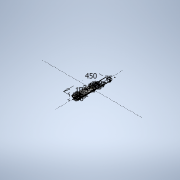
# Autodesk Inventor part: MoreFunComing-EnlosureEquipmentPanel
Saved by Autodesk Inventor 2021 (Build 250183000, 183)
## iProperties
Created: 2021-01-09
Part Number: MoreFunComing-EnlosureEquipmentPanel
Material: Generic
Document SubType Name: Modeling
Designer: incep
Density: 1 g/cm^3
Appearance: Default
Author: incep
Autodesk Inventor part; units mm, degrees
ref_plane "YZ Plane" through (0, 0, 0) normal (1, 0, 0) x (0, 1, 0)
ref_plane "XZ Plane" through (0, 0, 0) normal (0, 1, 0) x (-1, 0, 0)
ref_plane "XY Plane" through (0, 0, 0) normal (0, 0, 1) x (1, 0, 0)
sketch "Sketch1" plane through (0, 0, 0) normal (0, 1, 0) x (-1, 0, 0)
  line L0 (37.5, -225) -> (-37.5, -225)
  line L1 (-37.5, -225) -> (-37.5, 225)
  line L2 (-37.5, 225) -> (37.5, 225)
  line L3 (37.5, 225) -> (37.5, -225)
  line L4 (673.3706, 0) -> (-691.4675, 0) construction
  line L5 (0, 481.6336) -> (0, -423.6346) construction
  line L6 (31.5, -219) -> (-31.5, -219) construction
  line L7 (-31.5, -219) -> (-31.5, 219) construction
  line L8 (-31.5, 219) -> (31.5, 219) construction
  line L9 (31.5, 219) -> (31.5, -219) construction
  line L10 (34.5, -222) -> (-34.5, -222) construction
  line L11 (-34.5, -222) -> (-34.5, 222) construction
  line L12 (-34.5, 222) -> (34.5, 222) construction
  line L13 (34.5, 222) -> (34.5, -222) construction
  line L14 (14.5, 154.5) -> (-14.5, 154.5)
  line L15 (-14.5, 154.5) -> (-14.5, 211.5)
  line L16 (-14.5, 211.5) -> (14.5, 211.5)
  line L17 (14.5, 211.5) -> (14.5, 154.5)
  line L18 (50.1754, 183) -> (-68.7918, 183) construction
  circle A0 centre (20, 183) radius 1.5
  line L19 (0, 153.4917) -> (0, 241.4122) construction
  circle A1 centre (-20, 183) radius 1.5
  line L20 (25, 150) -> (-25, 150) construction
  line L21 (-25, 150) -> (-25, 216) construction
  line L22 (-25, 216) -> (25, 216) construction
  line L23 (25, 216) -> (25, 150) construction
  line L24 (27.05, 147) -> (-27.05, 147) construction
  line L25 (-27.05, 147) -> (-27.05, -44.4) construction
  line L26 (-27.05, -44.4) -> (27.05, -44.4) construction
  line L27 (27.05, -44.4) -> (27.05, 147) construction
  line L28 (-44.1096, 51.3) -> (44.1096, 51.3) construction
  line L29 (0, 385.9466) -> (0, -283.3466) construction
  circle A2 centre (12.7, -39.25) radius 2.4
  circle A3 centre (-12.7, -39.25) radius 2.4
  circle A4 centre (12.7, 141.85) radius 2.4
  circle A5 centre (-12.7, 141.85) radius 2.4
  line L30 (12.7, 141.85) -> (-12.7, 141.85) construction
  line L31 (-12.7, 141.85) -> (-12.7, -39.25) construction
  line L32 (-12.7, -39.25) -> (12.7, -39.25) construction
  line L33 (12.7, -39.25) -> (12.7, 141.85) construction
  line L34 (30, -47.4) -> (-30, -47.4) construction
  line L35 (-30, -47.4) -> (-30, -137.4) construction
  line L36 (-30, -137.4) -> (30, -137.4) construction
  line L37 (30, -137.4) -> (30, -47.4) construction
  circle A6 centre (12.7, -92.4) radius 2.4
  line L38 (34.7323, -92.4) -> (-30, -92.4) construction
  line L39 (0, -47.4) -> (0, -137.4) construction
  circle A7 centre (-12.7, -92.4) radius 2.4
  line L40 (51.05, 219) -> (-27.05, 219)
  line L41 (-27.05, 219) -> (-27.05, -44.4)
  line L42 (-27.05, -44.4) -> (51.05, -44.4)
  line L43 (51.05, -44.4) -> (51.05, 219)
  point P0 (0, 0)
  point P1 (-37.5, 0)
  point P2 (0, 225)
  point P3 (0, 154.5)
  point P4 (-14.5, 183)
  point P5 (-25, 183)
  point P6 (0, 216)
  point P7 (27.05, 51.3)
  point P8 (0, -44.4)
  point P9 (12.7, 51.3)
  point P10 (0, -39.25)
  point P11 (0, 51.3)
  point P12 (0, 51.3)
  point P13 (30, -92.4)
  dimension "d0" = 75
  dimension "d1" = 450
  dimension "d2" = 6
  dimension "d3" = 6
  dimension "d4" = 6
  dimension "d5" = 6
  dimension "d6" = 3
  dimension "d7" = 3
  dimension "d8" = 3
  dimension "d9" = 3
  dimension "d10" = 29
  dimension "d11" = 57
  dimension "d12" = 3
  dimension "d13" = 3
  dimension "d14" = 20
  dimension "d15" = 20
  dimension "d16" = 50
  dimension "d17" = 66
  dimension "d18" = 3
  dimension "d19" = 191.4
  dimension "d20" = 54.1
  dimension "d21" = 4.8
  dimension "d22" = 4.8
  dimension "d23" = 4.8
  dimension "d24" = 4.8
  dimension "d25" = 181.1
  dimension "d26" = 25.4
  dimension "d27" = 3
  dimension "d28" = 60
  dimension "d29" = 90
  dimension "d30" = 4.8
  dimension "d31" = 4.8
  dimension "d32" = 12.7
  dimension "d33" = 12.7
  dimension "d34" = 3
  dimension "d35" = 24
  constraints: 88 end point, 18 midpoint, 18 parallel, 16 point on line, 14 horizontal, 9 perpendicular, 8 centre point, 6 collinear, 4 coincident, 4 vertical
  measures "d0" distance of L0.start L0.end
  measures "d1" distance of L2.end L0.start
  measures "d2" distance between parallel lines of L1 L7
  measures "d3" distance between parallel lines of L2 L8
  measures "d4" distance between parallel lines of L3 L9
  measures "d5" distance between parallel lines of L0 L6
  measures "d6" distance between parallel lines of L1 L11
  measures "d7" distance between parallel lines of L0 L10
  measures "d8" distance between parallel lines of L3 L13
  measures "d9" distance between parallel lines of L2 L12
  measures "d10" distance of L14.start L14.end
  measures "d11" distance of L14.end L15.end
  measures "d12" diameter of A0
  measures "d13" diameter of A1
  measures "d14" distance from line of L19 A1.centre
  measures "d15" distance from line of L19 A0.centre
  measures "d16" distance of L20.start L20.end
  measures "d17" distance of L20.end L21.end
  measures "d18" distance between parallel lines of L8 L22
  measures "d19" distance of L26.end L24.start
  measures "d20" distance of L24.start L24.end
  measures "d21" diameter of A2
  measures "d22" diameter of A3
  measures "d23" diameter of A4
  measures "d24" diameter of A5
  measures "d25" distance of L32.end L30.start
  measures "d26" distance of L31.end L32.end
  measures "d27" distance between parallel lines of L24 L20
  measures "d28" distance of L34.start L34.end
  measures "d29" distance of L36.end L34.start
  measures "d30" diameter of A6
  measures "d31" diameter of A7
  measures "d32" distance from line of L39 A6.centre
  measures "d33" distance from line of L39 A7.centre
  measures "d34" distance between parallel lines of L26 L34
  measures "d35" distance between parallel lines of L27 L43
extrude "Extrusion1" add sketch "Sketch1" along normal blind 3 contours L42 L41 L40 L3 | L3 L40 L43 L42 | L14 L15 L16 L17 | A0 | A1 | A2 | A3 | A4 | A5
extrude "Extrusion2" cut sketch "Sketch1" along normal blind 3 contours L14 L15 L16 L17 | A0 | A1 | A2 | A3 | A4 | A5
body "Solid1"
